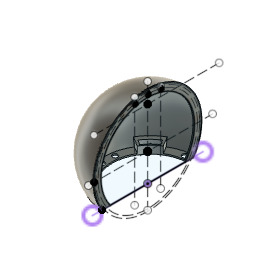
sphere2_dome v14 (Autodesk Fusion 360 design; units mm, degrees)
Autodesk Fusion 360 part; units mm, degrees
note: some values were not read from the file. Chosen so that the rebuilt part matches the saved one: which bodies a step acts on; a direction. Set by a fixed rule: which sketch regions a step uses.
sketch "Skizze1" plane through (0, 0, 0) normal (0, 0, 1) x (1, 0, 0)
  circle A0 centre (0, 0) radius 71.5
  circle A1 centre (0, 0) radius 69.5 construction
  line L0 (-102.9817, 0) -> (133.018, 0) construction
  line L1 (0, 78.3721) -> (0, -79.1293) construction
  line L2 (-59.4058, 59.4058) -> (72.0658, -72.0658) construction
  line L3 (76.6169, 76.6169) -> (-85.7695, -85.7695) construction
  line L4 (-54.193, 80.3445) -> (57.8444, -85.7578) construction
  line L5 (-70.58, 47.6068) -> (88.7008, -59.8295) construction
  line L6 (-79.2088, -53.427) -> (85.2644, 57.5116) construction
  line L7 (-48.526, -71.9428) -> (57.206, 84.8113) construction
  circle A2 centre (0, 0) radius 60.5 construction
  circle A3 centre (0, 0) radius 58.5
  arc A4 (-33.8312, 50.1568) -> (-50.1568, 33.8312) centre (0, 0) ccw
  arc A5 (-38.8639, 57.6181) -> (-57.6181, 38.8639) centre (0, 0) ccw
  arc A6 (-57.6181, -38.8639) -> (-38.8639, -57.6181) centre (0, 0) ccw
  arc A7 (-50.1568, -33.8312) -> (-33.8312, -50.1568) centre (0, 0) ccw
  line L8 (-33.8312, 50.1568) -> (-38.8639, 57.6181)
  line L9 (-50.1568, 33.8312) -> (-57.6181, 38.8639)
  line L10 (-33.8312, -50.1568) -> (-38.8639, -57.6181)
  line L11 (-50.1568, -33.8312) -> (-57.6181, -38.8639)
  line L12 (-43.202, -71.9002) -> (43.0491, 71.6457) construction
  line L13 (-71.6703, -43.0639) -> (80.1665, 48.1689) construction
  line L14 (-44.7415, 74.4623) -> (50.7143, -84.4028) construction
  line L15 (-71.3988, 42.9007) -> (82.9858, -49.8629) construction
  line L16 (-4, 71.388) -> (-4, -71.388)
  line L17 (-10, 81.1617) -> (-10, -106.0701) construction
  circle A8 centre (0, 0) radius 65 construction
  circle A9 centre (-10, 64.2262) radius 4.65
  circle A10 centre (-10, -64.2262) radius 4.65
  line L18 (-113.503, 10) -> (81.3894, 10) construction
  line L19 (-112.5836, -10) -> (93.1106, -10) construction
  circle A11 centre (-64.2262, 10) radius 4
  circle A12 centre (-64.2262, -10) radius 4
  line L20 (-50.1443, 30.1297) -> (-61.2875, 36.8252)
  line L21 (-30.1297, 50.1443) -> (-36.8252, 61.2875)
  line L22 (-50.1443, -30.1297) -> (-61.2875, -36.8252)
  line L23 (-30.1297, -50.1443) -> (-36.8252, -61.2875)
  line L24 (-77.5938, -35.5433) -> (-34.6617, -78.4754) construction
  line L25 (-81.6726, 31.4645) -> (-30.7659, 82.3712) construction
  line L26 (-4, -121.9343) -> (-4, -71.388)
  line L27 (-4, 71.388) -> (-4, 113.677)
  line L28 (-4, 113.677) -> (0, 113.677)
  line L29 (0, 113.677) -> (0, -121.9343)
  line L30 (0, -121.9343) -> (-4, -121.9343)
  point P0 (-33.8312, 50.1568)
  point P1 (-50.1568, 33.8312)
  point P2 (-57.6181, 38.8639)
  point P3 (-38.8639, 57.6181)
  point P4 (-33.8312, -50.1568)
  point P5 (-38.8639, -57.6181)
  point P6 (-57.6181, -38.8639)
  point P7 (-50.1568, -33.8312)
  point P8 (-30.1297, 50.1443)
  point P9 (-50.1443, 30.1297)
  point P10 (-50.1443, -30.1297)
  point P11 (-30.1297, -50.1443)
  point P12 (-61.2875, 36.8252)
  point P13 (-36.8252, 61.2875)
  point P14 (-61.2875, -36.8252)
  point P15 (-36.8252, -61.2875)
  point P16 (-10, -64.2262)
  point P17 (-10, 64.2262)
  dimension "d1" = 143
  dimension "d2" = 139
  dimension "d3" = 45
  dimension "d4" = 45
  dimension "d5" = 34
  dimension "d6" = 34
  dimension "d7" = 34
  dimension "d8" = 34
  dimension "d9" = 121
  dimension "d10" = 117
  dimension "d11" = 31
  dimension "d12" = 31
  dimension "d13" = 31
  dimension "d14" = 31
  dimension "d15" = 4
  dimension "d16" = 10
  dimension "d17" = 130
  dimension "d18" = 9.3
  dimension "d19" = 9.3
  dimension "d20" = 10
  dimension "d21" = 10
  dimension "d22" = 8
  dimension "d23" = 8
  dimension "d29" = 80
  dimension "d30" = 80
  constraint coincident A0.centre A1.centre
  constraint horizontal L0
  constraint coincident A0.centre L0
  constraint vertical L1
  constraint coincident A0.centre L1
  constraint coincident A0.centre L2
  constraint coincident A0.centre L3
  constraint coincident A0.centre L4
  constraint coincident A0.centre L5
  constraint coincident A0.centre L6
  constraint coincident A0.centre L7
  constraint coincident A2 P0
  constraint coincident L4 P0
  constraint coincident A2 P1
  constraint coincident L5 P1
  constraint coincident A1 P2
  constraint coincident L5 P2
  constraint coincident L4 P3
  constraint coincident A1 P3
  constraint coincident A2 P4
  constraint coincident L7 P4
  constraint coincident L7 P5
  constraint coincident A1 P5
  constraint coincident A1 P6
  constraint coincident L6 P6
  constraint coincident L6 P7
  constraint coincident A2 P7
  constraint coincident P0 A4.start
  constraint coincident P1 A4.end
  constraint coincident P3 A5.start
  constraint coincident P2 A5.end
  constraint coincident P6 A6.start
  constraint coincident P5 A6.end
  constraint coincident P7 A7.start
  constraint coincident P4 A7.end
  constraint coincident A0.centre L12
  constraint coincident A0.centre L13
  constraint coincident A0.centre L14
  constraint coincident A0.centre L15
  constraint coincident A3 P8
  constraint coincident L14 P8
  constraint coincident A3 P9
  constraint coincident L15 P9
  constraint coincident A3 P10
  constraint coincident L13 P10
  constraint coincident L12 P11
  constraint coincident A3 P11
  constraint coincident A0 P12
  constraint coincident L15 P12
  constraint coincident L14 P13
  constraint coincident A0 P13
  constraint coincident L13 P14
  constraint coincident A0 P14
  constraint coincident A0 P15
  constraint coincident L12 P15
  constraint vertical L16
  constraint coincident A0 L16.end
  constraint coincident A0 L16.start
  constraint vertical L17
  constraint coincident A8 P16
  constraint coincident L17 P16
  constraint coincident A8 P17
  constraint coincident L17 P17
  constraint coincident P17 A9.centre
  constraint coincident P16 A10.centre
  constraint horizontal L18
  constraint horizontal L19
  constraint coincident L18 A11.centre
  constraint coincident A8 A11.centre
  constraint coincident A8 A12.centre
  constraint coincident L19 A12.centre
  constraint coincident P9 L20.start
  constraint coincident P12 L20.end
  constraint coincident P8 L21.start
  constraint coincident P13 L21.end
  constraint coincident P10 L22.start
  constraint coincident P14 L22.end
  constraint coincident P11 L23.start
  constraint coincident P15 L23.end
  constraint perpendicular L3 L24
  constraint perpendicular L2 L25
  constraint parallel L17 L26
  constraint coincident L16.end L26.end
  constraint parallel L17 L27
  constraint coincident L16.start L27.start
  constraint perpendicular L27 L28
  constraint perpendicular L28 L29
  constraint perpendicular L26 L30
  constraint coincident L26.start L30.end
  measures "d1" diameter of A0
  measures "d2" diameter of A1
  measures "d3" angle of L0 L2
  measures "d4" angle of L0 L3
  measures "d5" angle of L0 L5
  measures "d6" angle of L1 L4
  measures "d7" angle of L0 L6
  measures "d8" angle of L1 L7
  measures "d9" diameter of A2
  measures "d10" diameter of A3
  measures "d11" angle of L1 L12
  measures "d12" angle of L0 L13
  measures "d13" angle of L1 L14
  measures "d14" angle of L0 L15
  measures "d15" distance of L1 L16
  measures "d16" distance of L1 L17
  measures "d17" diameter of A8
  measures "d18" diameter of A9
  measures "d19" diameter of A10
  measures "d20" distance of A0.centre L19
  measures "d21" distance of A0.centre L18
  measures "d22" diameter of A12
  measures "d23" diameter of A11
  measures "d29" distance of A0.centre L24
  measures "d30" distance of A0.centre L25
ref_plane "Arbeitsebene1" through (0, 0, 0) normal (0.707107, -0.707107, 0) x (0.707107, 0.707107, 0)
sketch "Skizze2" plane through (0, 0, 0) normal (0.707107, -0.707107, 0) x (0.707107, 0.707107, 0)
  line L0 (-80, 32.5981) -> (-80, -18.5904) construction
  dimension "d28" = 80
  constraint vertical L0
  measures "d28" distance of L0 origin
ref_plane "Arbeitsebene4" through (0, 0, 0) normal (0.707107, 0.707107, 0) x (-0.707107, 0.707107, 0)
sketch "Skizze9" plane through (0, 0, 0) normal (0.707107, 0.707107, 0) x (-0.707107, 0.707107, 0)
  line L0 (80, 27.3866) -> (80, -30.5152) construction
  dimension "d123" = 80
  constraint vertical L0
  measures "d123" distance of L0 origin
sketch "Skizze4" plane through (0, 0, 0) normal (1, 0, 0) x (0, 1, 0)
  line L0 (-85, 0) -> (85, 0) construction
  line L1 (0, 169.1462) -> (0, -34.5054) construction
  line L2 (-98.2939, 43) -> (93.2506, 43) construction
  line L3 (-71.5, 0) -> (-70.3305, 0)
  arc A0 (0, 126.4341) -> (-71.5, 0) centre (0, 43) ccw
  arc A1 (-82.4341, 43) -> (-70.3305, 0) centre (0, 43) ccw
  arc A2 (0, 125.4341) -> (-82.4341, 43) centre (0, 43) ccw
  line L4 (0, 125.4341) -> (0, 126.4341)
  line L5 (-69.5, 0) -> (-69.5, 12)
  line L6 (-76.3831, 12) -> (-69.5, 12)
  line L7 (-69.5, 0) -> (-70.3305, 0)
  point P0 (0, 43)
  point P1 (-83.4341, 43)
  point P2 (-82.4341, 43)
  dimension "d35" = 43
  dimension "d37" = 71.5
  dimension "d39" = 1
  dimension "d40" = 69.5
  dimension "d41" = 12
  constraint horizontal L0
  constraint coincident L0 origin
  constraint vertical L1
  constraint coincident origin L1
  constraint horizontal L2
  constraint horizontal L3
  constraint coincident origin L3
  constraint coincident L1 P0
  constraint coincident L2 P0
  constraint coincident L1 A0.start
  constraint coincident P0 A0.centre
  constraint coincident A0 P1
  constraint coincident L2 P1
  constraint coincident L2 P2
  constraint coincident L0 L3.end
  constraint coincident P2 A1.start
  constraint coincident L3.end A1
  constraint coincident L1 A2.start
  constraint vertical L5
  constraint coincident L0 L5.start
  constraint horizontal L6
  constraint coincident L5.end L6
  constraint coincident L5.end L6.end
  constraint coincident A1 L6.start
  measures "d35" distance of origin L2
  measures "d37" distance of L1 L3.start
  measures "d39" distance of P1 P2
  measures "d40" distance of origin L5
  measures "d41" distance of L0 L5.end
revolve "Drehen1" add sketch "Skizze4" angle 180 about axis through (0, 0, 169.1462) along (0, 0, -1) contours A1 L5 L6 L7 makes body 1
sketch "Skizze5" plane through (0, 0, 0) normal (0, 0, 1) x (1, 0, 0)
  line L0 (0, 95.2961) -> (0, -106.8691) construction
  line L1 (-90.7754, 0) -> (96.5619, 0) construction
  line L2 (-78.3947, 47.1043) -> (93.7935, -56.3568)
  line L3 (-102.9817, 0) -> (133.018, 0)
  line L4 (-55.1522, 91.7886) -> (51.5688, -85.825)
  line L5 (-47.9889, -79.8669) -> (54.3642, 90.4773)
  line L6 (-74.716, -44.8939) -> (89.049, 53.506)
  arc A0 (-72.8592, 43.7782) -> (-72.8592, -43.7782) centre (0, 0) ccw
  arc A1 (0, 85) -> (-43.7782, 72.8592) centre (0, 0) ccw
  line L7 (0, 0) -> (0, 85)
  arc A2 (-43.7782, -72.8592) -> (0, -85) centre (0, 0) ccw
  line L8 (0, 0) -> (0, -85)
  dimension "d43" = 31
  dimension "d44" = 31
  dimension "d45" = 31
  dimension "d46" = 31
  dimension "d47" = 85
  dimension "d48" = 85
  dimension "d49" = 85
  constraint vertical L0
  constraint coincident L0 A0.centre
  constraint horizontal L1
  constraint coincident L1 A0.centre
  constraint coincident L2 A0.centre
  constraint coincident A0.centre L4
  constraint coincident A0.centre L5
  constraint coincident A0.centre L6
  constraint coincident L2 A0.start
  constraint coincident L6 A0.end
  constraint coincident A0.centre A1.centre
  constraint coincident L0 A1.start
  constraint coincident L4 A1.end
  constraint coincident L0 A2.end
  constraint coincident L5 A2.start
  measures "d43" angle of L2 L3
  measures "d44" angle of L0 L4
  measures "d45" angle of L0 L5
  measures "d46" angle of L3 L6
  measures "d47" radius of A0
  measures "d48" radius of A1
  measures "d49" radius of A2
extrude "Extrusion4" cut sketch "Skizze5" along normal blind 20 bodies 1 makes body 2 at (-60.0668, -43.1094, 6.5454)
extrude "Extrusion5" add sketch "Skizze1" along normal blind 2 contours A0 A3 L16 L21 | A0 A3 L20 L21 | A0 A3 L20 L22 | A0 A3 L16 L23 | A0 A3 L22 L23 bodies 1 2
extrude "Extrusion6" add sketch "Skizze1" along normal blind 12 contours A0 A3 L20 L21 | A0 A3 L22 L23 bodies 1
revolve "Drehen2" add sketch "Skizze4" angle 180 about axis through (0, 0, 169.1462) along (0, 0, -1) contours L3 A0 A1 A2 L4 bodies 1
extrude "Extrusion7" cut sketch "Skizze1" along normal blind 200 contours A0 L27 L28 L29 | A0 A3 L16 L29 | A3 L16 L29 | A0 A3 L16 L29 | A0 L26 L29 L30 bodies 1
sketch "Skizze6" plane through (-4, 0, 0) normal (1, 0, 0) x (0, 1, 0)
  line L0 (71.388, 1.974) -> (71.388, 2)
  line L1 (71.388, 2) -> (58.3631, 2)
  line L2 (58.3631, 2) -> (58.3631, 0)
  line L3 (58.3631, 0) -> (71.388, 0)
  arc A0 (71.388, 0) -> (-71.388, 0) centre (0, 43) ccw
  line L4 (-71.388, 0) -> (-58.3631, 0)
  line L5 (-58.3631, 0) -> (-58.3631, 2)
  line L6 (-58.3631, 2) -> (-71.388, 2)
  line L7 (-71.388, 2) -> (-71.388, 1.974)
  arc A1 (71.388, 1.974) -> (-71.388, 1.974) centre (0, 43) ccw
  line L8 (-91.1854, 43) -> (100, 43) construction
  line L9 (0, 136.2962) -> (0, -35.4467) construction
  line L10 (-70.2167, 0) -> (70.2167, 0)
  arc A2 (-82.337, 43) -> (-70.2167, 0) centre (0, 43) ccw
  line L11 (-85, 0) -> (85, 0)
  arc A3 (70.2167, 0) -> (-82.337, 43) centre (0, 43) ccw
  arc A4 (57.7495, 0) -> (-57.7495, 0) centre (0, 43) ccw
  line L12 (20, 119.9802) -> (20, -16.5008) construction
  line L13 (-20, 125.337) -> (-20, -18.7847) construction
  line L14 (-82.6817, 106) -> (110, 106) construction
  circle A5 centre (0, 106) radius 3.75
  circle A6 centre (0, 43) radius 76.5 construction
  circle A7 centre (0, 43) radius 80 construction
  point P0 (0, 43)
  point P1 (-82.337, 43)
  point P2 (0, 106)
  point P3 (-20, 116.8394)
  point P4 (0, 119.5)
  point P5 (20, 116.8394)
  dimension "d59" = 43
  dimension "d60" = 72
  dimension "d88" = 20
  dimension "d89" = 20
  dimension "d140" = 82.337
  dimension "d154" = 63
  dimension "d155" = 7.5
  dimension "d161" = 153
  dimension "d167" = 160
  constraint horizontal L8
  constraint vertical L9
  constraint coincident L9 P0
  constraint coincident A1 P1
  constraint coincident L8 P1
  constraint horizontal L10
  constraint coincident origin L10
  constraint coincident L4 L10.start
  constraint coincident P1 A2.start
  constraint coincident P0 A0.centre
  constraint coincident L10.start A2.end
  constraint coincident L10 A3.start
  constraint coincident L10.end A3.start
  constraint coincident L10 A4.start
  constraint coincident L10 A4.end
  constraint vertical L12
  constraint vertical L13
  constraint horizontal L14
  constraint coincident L9 P2
  constraint coincident L14 P2
  constraint coincident P2 A5.centre
  constraint coincident A6 P3
  constraint coincident L13 P3
  constraint coincident A6 P4
  constraint coincident L9 P4
  constraint coincident A6 P5
  constraint coincident L12 P5
  measures "d59" distance of L8 origin
  measures "d60" radius of A4
  measures "d88" distance of P0 L12
  measures "d89" distance of P0 L13
  measures "d140" radius of A3
  measures "d154" distance of P0 L14
  measures "d155" diameter of A5
  measures "d161" diameter of A6
  measures "d167" diameter of A7
extrude "Extrusion8" add sketch "Skizze6" against normal blind 2 contours L0 L1 L6 L7 A1 A2 A3 A4 bodies 1
ref_plane "Arbeitsebene5" through (-56.5685, -56.5685, 0) normal (0.707107, 0.707107, 0) x (-0.707107, 0.707107, 0)
sketch "Skizze10" plane through (-56.5685, -56.5685, 0) normal (0.707107, 0.707107, 0) x (-0.707107, 0.707107, 0)
  line L0 (28.8531, 5) -> (-35.6558, 5) construction
  line L1 (0, 28.2666) -> (0, -28.2666) construction
  circle A0 centre (0, 5) radius 1.75
  circle A1 centre (0, 5) radius 4
  dimension "d124" = 5
  dimension "d125" = 3.5
  dimension "d127" = 8
  constraint horizontal L0
  constraint vertical L1
  constraint coincident origin L1
  constraint coincident L1 A0.centre
  constraint coincident L0 A0.centre
  constraint concentric A0 A1
  measures "d124" distance of L0 origin
  measures "d125" diameter of A0
  measures "d127" diameter of A1
extrude "Extrusion15" cut sketch "Skizze10" along normal blind 30 contours A0 bodies 1
extrude "Extrusion16" cut sketch "Skizze10" along normal blind 8 bodies 1
ref_plane "Arbeitsebene6" through (-56.5685, 56.5685, 0) normal (0.707107, -0.707107, 0) x (0.707107, 0.707107, 0)
sketch "Skizze11" plane through (-56.5685, 56.5685, 0) normal (0.707107, -0.707107, 0) x (0.707107, 0.707107, 0)
  line L0 (0, 14.8058) -> (0, -30) construction
  line L1 (22.7945, 5) -> (-30, 5) construction
  circle A0 centre (0, 5) radius 1.75
  circle A1 centre (0, 5) radius 4
  dimension "d132" = 5
  dimension "d133" = 3.5
  dimension "d134" = 8
  constraint vertical L0
  constraint coincident L0 origin
  constraint horizontal L1
  constraint coincident L1 A0.centre
  constraint coincident L0 A0.centre
  constraint concentric A0 A1
  measures "d132" distance of origin L1
  measures "d133" diameter of A0
  measures "d134" diameter of A1
extrude "Extrusion17" cut sketch "Skizze11" along normal blind 30 contours A0 bodies 1
extrude "Extrusion18" cut sketch "Skizze11" along normal blind 8 bodies 1
hole "Bohrung2" at (-4, -20, 116.8394) at (-4, 0, 119.5) at (-4, 20, 116.8394) direction (-1, 0, 0) diameter 3.5 depth 15 tip angle 90 countersink diameter 6 countersink angle 90 bodies 1
equation "d37 = ( 143 / 2 ) * 1 mm"
